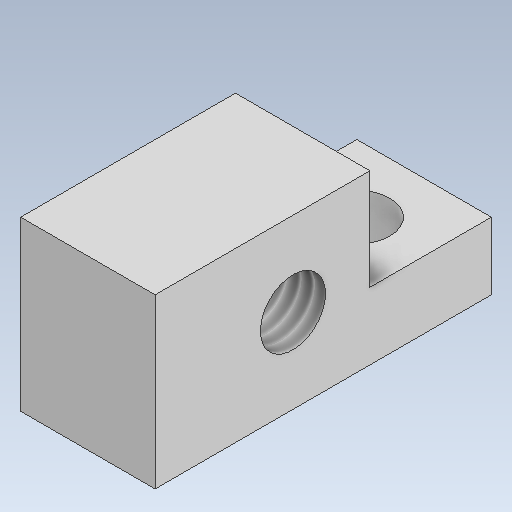
# Autodesk Inventor part: filament holders
Saved by Autodesk Inventor 2020 (Build 240168000, 168)
## iProperties
Created: 2019-06-14
Part Number: filament holders
Material: Generic
Document SubType Name: Modeling
Designer: ColinP
Density: 1 g/cm^3
Appearance: Default
Mass: 0.284458 g
Surface Area: 3.59769 cm^2
Volume: 0.284458 cm^3
Author: ColinP
Autodesk Inventor part; units mm, degrees
ref_plane "YZ Plane" through (0, 0, 0) normal (1, 0, 0) x (0, 1, 0)
ref_plane "XZ Plane" through (0, 0, 0) normal (0, 1, 0) x (-1, 0, 0)
ref_plane "XY Plane" through (0, 0, 0) normal (0, 0, 1) x (1, 0, 0)
sketch "Sketch20" plane through (0, 0, 0) normal (0, 1, 0) x (-1, 0, 0)
  line L0 (1.5185, -0.8925) -> (-3.5615, -0.8925)
  line L1 (-3.5615, -0.8925) -> (-3.5615, 11.8075)
  line L2 (-3.5615, 11.8075) -> (1.5185, 11.8075)
  line L3 (1.5185, 11.8075) -> (1.5185, -0.8925)
  line L4 (1.5185, 4.9634) -> (-3.5615, 4.9634)
  point P0 (0, 0)
  dimension "d56" = 5.08
  dimension "d57" = 12.7
  constraints: 10 end point, 2 parallel, 2 perpendicular, 2 point on line, 1 horizontal
  measures "d56" distance of L1.end L2.end
  measures "d57" distance of L0.end L1.end
extrude "Extrusion7" add sketch "Sketch20" along normal blind 2.54 contours L0 L1 L4 L3
extrude "Extrusion8" add sketch "Sketch20" along normal blind 6.35 contours L4 L1 L2 L3
sketch "Sketch21" plane through (0, 2.54, 0) normal (0, 1, 0) x (1, 0, 0)
  line L0 (3.5615, 0.8925) -> (-1.5185, 0.8925) projected
  line L1 (-1.5185, 0.8925) -> (-1.5185, -4.9634) projected
  point P0 (0, 0)
  point P1 (1.0215, -1.6475)
  dimension "d62" = 2.54
  dimension "d63" = 2.54
  measures "d62" distance from line of L0 point (1.021, -1.648)
  measures "d63" distance from line of L1 point (1.021, -1.648)
hole "Hole5" at (1.0215, 2.54, 1.6475) direction (0, -1, 0) diameter 2.4867 end through all
sketch "Sketch22" plane through (3.5615, 0, -0.8925) normal (1, 0, 0) x (0, 0, -1)
  line L0 (-12.7, 6.35) -> (-5.8558, 6.35) projected
  line L1 (-12.7, 0) -> (-12.7, 6.35) projected
  point P0 (-0.8925, 0)
  point P1 (-7.493, 3.175)
  dimension "d71" = 3.175
  dimension "d72" = 5.207
  measures "d71" distance from line of L0 point (-7.493, 3.175)
  measures "d72" distance from line of L1 point (-7.493, 3.175)
hole "Hole6" at (3.5615, 3.175, 6.6005) direction (-1, 0, 0) diameter 2.459 end through all thread size "M3x0.5" class "6H" standard "ISO Metric profile"
sketch "Sketch23" plane through (0, 2.54, 0) normal (0, 1, 0) x (1, 0, 0)
  line L0 (-1.5185, 0.8925) -> (-1.5185, -4.9634) projected
  line L1 (-1.5185, -4.9634) -> (-1.5185, -3.6934)
  line L2 (-1.5185, -3.6934) -> (3.5615, -3.6934)
  line L3 (3.5615, -4.9634) -> (3.5615, 0.8925) projected
  line L4 (3.5615, -3.6934) -> (3.5615, -4.9634)
  line L5 (3.5615, -11.8075) -> (3.5615, 0.8925) projected
  line L6 (3.5615, -4.9634) -> (-1.5185, -4.9634) projected
  line L7 (-1.5185, -4.9634) -> (3.5615, -4.9634)
  point P0 (0, 0)
  dimension "d80" = 1.27
  constraints: 8 end point, 3 point on line, 2 perpendicular
  measures "d80" distance of L0.end L1.end
extrude "Extrusion9" add sketch "Sketch23" along normal blind 3.81
body "Solid2"
